Autodesk Fusion 360 part; units mm, degrees
note: some values were not read from the file. Chosen so that the rebuilt part matches the saved one: which face or edge a step refers to; a direction. Set by a fixed rule: which sketch regions a step uses.
(part 2 of 2)
copy_body "CopyPasteBodies18" bodies 51 52 makes body 53 makes body 54
move_body "Move24" bodies 53 54 to x (1, 0, 0) y (0, 1, 0) z (0, 0, 1) at (0, 0, 2.85)
copy_body "CopyPasteBodies19" bodies 51 52 53 54 makes body 55 makes body 56 makes body 57 makes body 58
move_body "Move25" bodies 55 56 57 58 to x (1, 0, 0) y (0, 1, 0) z (0, 0, 1) at (0, 0, 5)
copy_body "CopyPasteBodies20" bodies 51 52 53 54 55 56 57 58 makes body 59 makes body 60 makes body 61 makes body 62 makes body 63 makes body 64 makes body 65 makes body 66
move_body "Move26" bodies 59 60 61 62 63 64 65 66 to x (1, 0, 0) y (0, 1, 0) z (0, 0, 1) at (0, 0, -10.5)
move_body "Move27" bodies 58 57 to x (1, 0, 0) y (0, 1, 0) z (0, 0, 1) at (0, 0, -0.4)
extrude "Extrude25" add 1 faces at (5.7503, 0, 5.5348) along direction (0, -1, 0) blind 0.1 separate body on bodies 1 makes body 67
component "Component" placed x (1, 0, 0) y (0, 1, 0) z (0, 0, 1) at (0, 0, 0)
component "Component" placed x (1, 0, 0) y (0, 1, 0) z (0, 0, 1) at (7.1877, 0.1427, -14.6977)
component "Component''" placed x (1, 0, 0) y (0, 1, 0) z (0, 0, 1) at (0, 0, 0)
component "Component'''" placed x (1, 0, 0) y (0, 1, 0) z (0, 0, 1) at (0, 0, 0)
component "Component''''" placed x (1, 0, 0) y (0, 1, 0) z (0, 0, 1) at (0, 0, 0)
component "Component'''''" placed x (1, 0, 0) y (0, 1, 0) z (0, 0, 1) at (0, 0, 0)
component "Component''''''" placed x (1, 0, 0) y (0, 1, 0) z (0, 0, 1) at (0, 0, 0)
component "Component''" placed x (-1, 0, 0) y (0, 1, 0) z (0, 0, -1) at (-13.3695, 0, -0.2981)
component "Component'''''" placed x (-1, 0, 0) y (0, 1, 0) z (0, 0, -1) at (-13.3695, 0, -0.2981)
component "Component''''''" placed x (-1, 0, 0) y (0, 1, 0) z (0, 0, -1) at (-13.3695, 0, -0.2981)
component "Component'''" placed x (-1, 0, 0) y (0, 1, 0) z (0, 0, -1) at (-13.3695, 0, -0.2981)
component "Component''''" placed x (-1, 0, 0) y (0, 1, 0) z (0, 0, -1) at (-13.3695, 0, -0.2981)
component "Component''" placed x (-1, 0, 0) y (0, 1, 0) z (0, 0, -1) at (-26.8695, 0, 4.0019)
component "Component''" placed x (-1, 0, 0) y (0, 1, 0) z (0, 0, -1) at (-26.7695, 0, 9.1019)
component "Component''" placed x (-1, 0, 0) y (0, 1, 0) z (0, 0, -1) at (-26.7695, 0, 14.1019)
component "Component''''" placed x (0, 0, 1) y (0, 1, 0) z (-1, 0, 0) at (0.3833, -0.3, -9.2546)
component "Component''''" placed x (0, 0, 1) y (0, 1, 0) z (-1, 0, 0) at (0.3833, -0.3, -4.2546)
component "Component''''" placed x (0, 0, 1) y (0, 1, 0) z (-1, 0, 0) at (0.3833, -0.3, 0.4454)
component "Component'" placed x (1, 0, 0) y (0, 1, 0) z (0, 0, 1) at (0, 0, 0) in component "Component"

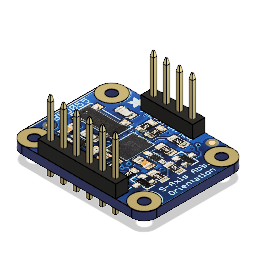
design "BNO055 gyroscope"
Autodesk Fusion 360 part; units mm, degrees
sketch "Sketch1" plane through (0, 0, 0) normal (0, 1, 0) x (1, 0, 0)
  line L0 (0, 0) -> (27, 0)
  line L1 (27, 0) -> (27, 20.5)
  line L2 (27, 20.5) -> (0, 20.5)
  line L3 (0, 20.5) -> (0, 0)
  circle A0 centre (2.5, 17.9984) radius 1
  line L4 (27, 19) -> (1.5, 19)
  line L5 (1.5, 19) -> (1.5, 0)
  line L6 (2.4988, 18.9984) -> (2.4988, 16.9984)
  line L7 (3.5, 17.9991) -> (1.5, 17.9991)
  circle A1 centre (2.5, 17.9984) radius 2.5
  line L8 (2.4988, 18.9984) -> (2.4988, 20.5)
  line L9 (1.5, 17.9991) -> (0, 18)
  line L10 (0, 10.25) -> (27, 10.25)
  line L11 (13.5, 0) -> (13.5, 20.5)
  circle A2 centre (24.5, 17.9984) radius 1
  line L12 (24.5012, 18.9984) -> (24.5012, 20.5)
  line L13 (25.5, 17.9991) -> (27, 18)
  circle A3 centre (24.5, 17.9984) radius 2.5
  line L14 (25.5, 19) -> (25.5, 0)
  line L15 (25.5, 2.5009) -> (27, 2.5)
  circle A4 centre (24.5, 2.5016) radius 2.5
  line L16 (24.5012, 1.5016) -> (24.5012, 0)
  circle A5 centre (2.5, 2.5016) radius 1
  line L17 (27, 1.5) -> (1.5, 1.5)
  circle A6 centre (2.5, 2.5016) radius 2.5
  line L18 (2.4988, 1.5016) -> (2.4988, 0)
  line L19 (1.5, 2.5009) -> (0, 2.5)
  circle A7 centre (24.5, 2.5016) radius 1
  line L20 (0, 20.5) -> (18.7, 20.5)
  line L21 (27, 20.5) -> (8.3, 20.5)
  line L22 (8.3, 20.5) -> (18.7, 20.5)
  line L23 (18.7, 20.5) -> (18.7, 18)
  line L24 (18.7, 18) -> (8.3, 18)
  line L25 (8.3, 18) -> (8.3, 20.5)
  line L26 (8.3, 20.5) -> (18.7, 20.5)
  line L27 (8.3, 20.5) -> (10.9, 20.5)
  line L28 (10.9, 20.5) -> (10.9, 18)
  line L29 (8.3, 19.25) -> (18.7, 19.25)
  line L30 (18.7, 20.5) -> (16.1, 20.5)
  line L31 (16.1, 20.5) -> (16.1, 18)
  line L32 (9.25, 19.6) -> (9.95, 19.6)
  line L33 (9.95, 19.6) -> (9.95, 18.9)
  line L34 (9.95, 18.9) -> (9.25, 18.9)
  line L35 (9.25, 18.9) -> (9.25, 19.6)
  line L36 (9.6, 19.6) -> (9.6, 18.9)
  line L37 (9.25, 19.25) -> (9.95, 19.25)
  line L38 (9.6, 20.5) -> (9.6, 18)
  line L39 (11.85, 19.25) -> (12.55, 19.25)
  line L40 (12.55, 18.9) -> (11.85, 18.9)
  line L41 (12.2, 19.6) -> (12.2, 18.9)
  line L42 (11.85, 19.6) -> (12.55, 19.6)
  line L43 (11.85, 18.9) -> (11.85, 19.6)
  line L44 (12.55, 19.6) -> (12.55, 18.9)
  line L45 (15.15, 19.6) -> (15.15, 18.9)
  line L46 (14.8, 19.6) -> (14.8, 18.9)
  line L47 (15.15, 18.9) -> (14.45, 18.9)
  line L48 (14.45, 19.6) -> (15.15, 19.6)
  line L49 (17.05, 19.25) -> (17.75, 19.25)
  line L50 (14.45, 19.25) -> (15.15, 19.25)
  line L51 (14.45, 18.9) -> (14.45, 19.6)
  line L52 (17.4, 19.6) -> (17.4, 18.9)
  line L53 (17.75, 18.9) -> (17.05, 18.9)
  line L54 (17.05, 18.9) -> (17.05, 19.6)
  line L55 (17.75, 19.6) -> (17.75, 18.9)
  line L56 (17.05, 19.6) -> (17.75, 19.6)
  dimension "d57" = 20.5
  dimension "d58" = 27
  dimension "d59" = 2
  dimension "d60" = -1.5
  dimension "d61" = 1.5
  dimension "d66" = 18.7
  dimension "d67" = 18.7
  dimension "d68" = 2.5
  dimension "d69" = 2.6
  dimension "d70" = 2.6
  dimension "d71" = 0.7
  dimension "d72" = 0.7
  dimension "d73" = 0.7
  dimension "d74" = 0.7
  dimension "d75" = 0.7
  dimension "d76" = 0.7
  dimension "d77" = 0.7
  dimension "d78" = 0.7
  measures "d59" diameter of A0
  measures "d66" distance of L0.start
  measures "d67" distance of L0.start
extrude "Extrude4" add sketch "Sketch1" along normal blind 10.3 contours L29 L32 L35 L36 L37 L38 | L29 L32 L33 L36 L37 L38 | L4 L29 L35 L36 L37 L38 | L4 L34 L35 L36 L38 | L4 L29 L46 L50 L51 | L4 L46 L47 L51 | L4 L40 L41 L44 | L4 L29 L39 L41 L44 | L4 L29 L33 L36 L37 L38 | L4 L33 L34 L36 L38 | L4 L29 L45 L46 L50 | L4 L45 L46 L47 | L29 L46 L48 L50 L51 | L4 L40 L41 L43 | L4 L29 L39 L41 L43 | L29 L39 L41 L42 L44 | L4 L29 L49 L52 L54 | L4 L52 L53 L54 | L29 L39 L41 L42 L43 | L4 L52 L53 L55 | L4 L29 L49 L52 L55 | L29 L45 L46 L48 L50 | L29 L49 L52 L54 L56 | L29 L49 L52 L55 L56 makes body 1 at (14.6833, 3.4333, -19.6) makes body 2 at (17.75, 3.4333, -19.3667) makes body 3 at (11.85, 3.4333, -19.1333) makes body 4 at (9.7167, 3.4333, -18.9)
extrude "Extrude1" add sketch "Sketch1" against normal blind 1.7 separate body contours L3 L5 L10 A6 | L5 A1 L9 | L5 A6 L19 | L5 A5 L17 A6 | L5 A6 L19 | L0 L11 L17 A6 | L17 A6 L18 | L5 L17 A6 L18 | L4 L5 A1 L8 L9 | L3 L5 A1 L10 | L5 L10 L11 L17 A6 | L5 A5 L17 | L0 L11 A4 L17 | L4 L5 A1 L10 L11 L24 L25 | L14 A4 L16 L17 | A4 L16 L17 | L10 L11 L14 A4 L17 | L2 L4 A1 L20 L25 | L4 A1 L8 | L4 L5 A1 | L4 L10 L11 A3 L14 L23 L24 | L14 A4 L17 A7 | L14 A4 L17 | L14 L17 A7 | L2 L20 L21 L22 L25 L26 L27 L29 L32 L35 L38 | L1 L10 A3 L14 | L1 L10 L14 A4 | L4 L11 L24 L28 L40 L43 L44 | L4 L11 L24 L31 L45 L47 L51 | L14 L15 A4 | L14 L15 A4 L17 | L2 L20 L21 L22 L26 L27 L28 L29 L32 L33 L38 | L4 L25 L29 L35 | L4 L24 L25 L34 L35 L38 | L13 A3 L14 | L4 A2 A3 L14 | L4 L11 L29 L51 | L4 L11 L29 L44 | L4 L23 L24 L31 L53 L54 L55 | L4 L24 L28 L33 L34 L38 | L2 L11 L20 L21 L22 L26 L28 L29 L42 L43 L44 | L29 L32 L35 L36 L37 L38 | L29 L32 L33 L36 L37 L38 | L4 L29 L35 L36 L37 L38 | L4 L34 L35 L36 L38 | L4 L13 A3 L14 | L4 L12 A3 | L2 L4 A3 L21 L23 | L4 A2 L14 | L4 L29 L46 L50 L51 | L4 L46 L47 L51 | L4 L40 L41 L44 | L4 L29 L39 L41 L44 | L2 L11 L20 L21 L22 L26 L29 L31 L45 L48 L51 | L4 L29 L31 L54 | L4 L29 L31 L45 | L4 L28 L29 L43 | L4 L28 L29 L33 | L4 L29 L33 L36 L37 L38 | L4 L33 L34 L36 L38 | L4 L12 A3 | L4 L23 L29 L55 | L4 L29 L45 L46 L50 | L4 L45 L46 L47 | L29 L46 L48 L50 L51 | L4 L40 L41 L43 | L4 L29 L39 L41 L43 | L29 L39 L41 L42 L44 | L4 L29 L49 L52 L54 | L4 L52 L53 L54 | L2 L20 L21 L22 L23 L26 L29 L30 L31 L54 L55 L56 | L29 L39 L41 L42 L43 | L4 L52 L53 L55 | L4 L29 L49 L52 L55 | L29 L45 L46 L48 L50 | L29 L49 L52 L54 L56 | L29 L49 L52 L55 L56 makes body 5
extrude "Extrude2" add sketch "Sketch1" against normal blind 0.1 separate body contours L5 A1 L9 | L5 A6 L19 | L5 A5 L17 A6 | L5 A6 L19 | L17 A6 L18 | L5 L17 A6 L18 | L4 L5 A1 L8 L9 | L5 A5 L17 | L14 A4 L16 L17 | A4 L16 L17 | L4 A1 L8 | L4 L5 A1 | L14 A4 L17 A7 | L14 A4 L17 | L14 L17 A7 | L14 L15 A4 | L14 L15 A4 L17 | L13 A3 L14 | L4 A2 A3 L14 | L4 L13 A3 L14 | L4 L12 A3 | L4 A2 L14 | L4 L12 A3 makes body 6 at (25.1765, 0, -16.1217) makes body 7 at (25.1765, 0, -4.3783) makes body 8 at (1.8502, 0, -16.1117) makes body 9 at (2.946, 0, -4.447)
combine "Combine1" operation cut target body 5 tool bodies 7 8 6 9 keep tools
extrude "Extrude3" add sketch "Sketch1" along normal blind 2.6 separate body contours L2 L20 L21 L22 L25 L26 L27 L29 L32 L35 L38 | L4 L11 L24 L28 L40 L43 L44 | L4 L11 L24 L31 L45 L47 L51 | L2 L20 L21 L22 L26 L27 L28 L29 L32 L33 L38 | L4 L25 L29 L35 | L4 L24 L25 L34 L35 L38 | L4 L11 L29 L51 | L4 L11 L29 L44 | L4 L23 L24 L31 L53 L54 L55 | L4 L24 L28 L33 L34 L38 | L2 L11 L20 L21 L22 L26 L28 L29 L42 L43 L44 | L29 L32 L35 L36 L37 L38 | L29 L32 L33 L36 L37 L38 | L4 L29 L35 L36 L37 L38 | L4 L34 L35 L36 L38 | L4 L29 L46 L50 L51 | L4 L46 L47 L51 | L4 L40 L41 L44 | L4 L29 L39 L41 L44 | L2 L11 L20 L21 L22 L26 L29 L31 L45 L48 L51 | L4 L29 L31 L54 | L4 L29 L31 L45 | L4 L28 L29 L43 | L4 L28 L29 L33 | L4 L29 L33 L36 L37 L38 | L4 L33 L34 L36 L38 | L4 L23 L29 L55 | L4 L29 L45 L46 L50 | L4 L45 L46 L47 | L29 L46 L48 L50 L51 | L4 L40 L41 L43 | L4 L29 L39 L41 L43 | L29 L39 L41 L42 L44 | L4 L29 L49 L52 L54 | L4 L52 L53 L54 | L2 L20 L21 L22 L23 L26 L29 L30 L31 L54 L55 L56 | L29 L39 L41 L42 L43 | L4 L52 L53 L55 | L4 L29 L49 L52 L55 | L29 L45 L46 L48 L50 | L29 L49 L52 L54 L56 | L29 L49 L52 L55 L56 makes body 10
extrude "Extrude5" add sketch "Sketch1" 4 faces at (17.2833, 0, -19.3667) (14.6833, 0, -19.3667) (12.3167, 0, -19.3667) (9.7167, 0, -19.3667) along normal blind 3.7 contours L29 L32 L35 L36 L37 L38 | L29 L32 L33 L36 L37 L38 | L4 L29 L35 L36 L37 L38 | L4 L34 L35 L36 L38 | L4 L29 L46 L50 L51 | L4 L46 L47 L51 | L4 L40 L41 L44 | L4 L29 L39 L41 L44 | L4 L29 L33 L36 L37 L38 | L4 L33 L34 L36 L38 | L4 L29 L45 L46 L50 | L4 L45 L46 L47 | L29 L46 L48 L50 L51 | L4 L40 L41 L43 | L4 L29 L39 L41 L43 | L29 L39 L41 L42 L44 | L4 L29 L49 L52 L54 | L4 L52 L53 L54 | L29 L39 L41 L42 L43 | L4 L52 L53 L55 | L4 L29 L49 L52 L55 | L29 L45 L46 L48 L50 | L29 L49 L52 L54 L56 | L29 L49 L52 L55 L56 on bodies 1 2 3 4 bodies 2 1 3 4
extrude "Extrude6" add sketch "Sketch1" 4 faces at (9.7167, 0, -19.3667) (12.3167, 0, -19.3667) (14.6833, 0, -19.3667) (17.2833, 0, -19.3667) against normal blind 3.7 contours L29 L32 L35 L36 L37 L38 | L29 L32 L33 L36 L37 L38 | L4 L29 L35 L36 L37 L38 | L4 L34 L35 L36 L38 | L4 L29 L46 L50 L51 | L4 L46 L47 L51 | L4 L40 L41 L44 | L4 L29 L39 L41 L44 | L4 L29 L33 L36 L37 L38 | L4 L33 L34 L36 L38 | L4 L29 L45 L46 L50 | L4 L45 L46 L47 | L29 L46 L48 L50 L51 | L4 L40 L41 L43 | L4 L29 L39 L41 L43 | L29 L39 L41 L42 L44 | L4 L29 L49 L52 L54 | L4 L52 L53 L54 | L29 L39 L41 L42 L43 | L4 L52 L53 L55 | L4 L29 L49 L52 L55 | L29 L45 L46 L48 L50 | L29 L49 L52 L54 L56 | L29 L49 L52 L55 L56 on bodies 1 2 3 4 bodies 4 1 2 3
chamfer "Chamfer1" distance 0.2 distance2 1 4 edges at (17.75, 10.3, -19.25) (17.4, 10.3, -19.6) (17.4, 10.3, -18.9) (17.05, 10.3, -19.25) measured on face at (17.2833, 10.3, -19.3667) measured on face at (17.2833, 10.3, -19.3667) measured on face at (17.2833, 10.3, -19.3667) measured on face at (17.2833, 10.3, -19.3667) on bodies 2
chamfer "Chamfer2" distance 0.2 distance2 1 4 edges at (14.8, 10.3, -19.6) (14.45, 10.3, -19.25) (14.8, 10.3, -18.9) (15.15, 10.3, -19.25) measured on face at (14.6833, 10.3, -19.3667) measured on face at (14.6833, 10.3, -19.3667) measured on face at (14.6833, 10.3, -19.3667) measured on face at (14.6833, 10.3, -19.3667) on bodies 1
chamfer "Chamfer3" distance 0.2 distance2 1 4 edges at (12.55, 10.3, -19.25) (12.2, 10.3, -18.9) (11.85, 10.3, -19.25) (12.2, 10.3, -19.6) measured on face at (12.3167, 10.3, -19.3667) measured on face at (12.3167, 10.3, -19.3667) measured on face at (12.3167, 10.3, -19.3667) measured on face at (12.3167, 10.3, -19.3667) on bodies 3
chamfer "Chamfer4" distance 0.2 distance2 1 4 edges at (9.6, 10.3, -19.6) (9.95, 10.3, -19.25) (9.6, 10.3, -18.9) (9.25, 10.3, -19.25) measured on face at (9.7167, 10.3, -19.3667) measured on face at (9.7167, 10.3, -19.3667) measured on face at (9.7167, 10.3, -19.3667) measured on face at (9.7167, 10.3, -19.3667) on bodies 4
copy_body "CopyPasteBodies1" bodies 10 makes body 11
move_body "Move1" bodies 11 to x (1, 0, 0) y (0, 1, 0) z (0, 0, 1) at (0, 0, 18)
extrude "Extrude7" add 3 faces at (8.3, 0.8667, -1.0833) (8.3, 0.8667, -0.3333) (8.3, 0.8667, -1.6667) along direction (-1, 0, 0) blind 2.6 on bodies 11 bodies 11
extrude "Extrude8" add 1 faces at (18.7, 0.8667, -1.6667) along direction (1, 0, 0) blind 2.6 on bodies 11 bodies 11
copy_body "CopyPasteBodies2" bodies 1 3 4 2 makes body 12 makes body 13 makes body 14 makes body 15
move_body "Move2" bodies 12 13 14 15 to x (1, 0, 0) y (0, 1, 0) z (0, 0, 1) at (0, 0, 18)
copy_body "CopyPasteBodies3" bodies 15 makes body 16
move_body "Move3" bodies 16 to x (1, 0, 0) y (0, 1, 0) z (0, 0, 1) at (2.6, 0, 0)
copy_body "CopyPasteBodies5" bodies 14 makes body 17
move_body "Move5" bodies 17 to x (1, 0, 0) y (0, 1, 0) z (0, 0, 1) at (-2.6, 0, 0)
equation "d79 = 4.3 mm - 1.7 mm"
equation "d83 = -1.7 mm - 2 mm"
equation "d95 = ( 10.4 / 4 ) * 1 mm"
equation "d97 = ( 10.4 / 4 ) * 1 mm"
named bodies: "board"
